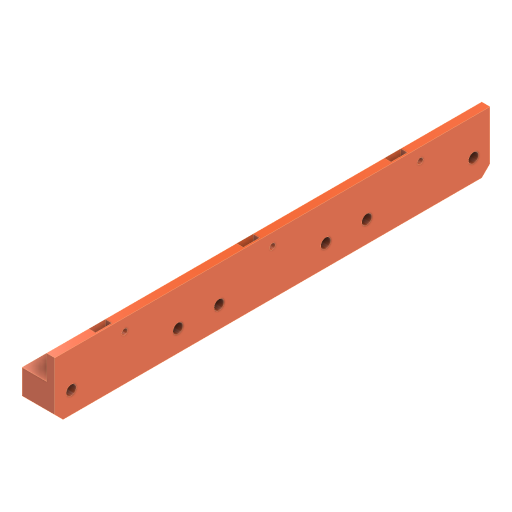
# Autodesk Inventor part: Toolhead Dock Assembly
Saved by Autodesk Inventor 2023.2 (Build 272271000, 271)
## iProperties
Created: 2023-02-06
Part Number: Toolhead Dock Assembly
Material: ABS Plastic
Document SubType Name: Modeling
Designer: remop
Density: 1.06 g/cm^3
Appearance: Smooth - Light Orange
Author: remop
Autodesk Inventor part; units mm, degrees
ref_plane "YZ Plane" through (0, 0, 0) normal (1, 0, 0) x (0, 1, 0)
ref_plane "XZ Plane" through (0, 0, 0) normal (0, 1, 0) x (-1, 0, 0)
ref_plane "XY Plane" through (0, 0, 0) normal (0, 0, 1) x (1, 0, 0)
sketch "Sketch1" plane through (0, 0, 0) normal (0, 0, 1) x (1, 0, 0)
  line L0 (0, 0) -> (0, 15)
  line L1 (0, 15) -> (5, 15)
  line L2 (5, 15) -> (5, -20)
  line L3 (5, -20) -> (-15, -20)
  line L4 (-15, -20) -> (-15, 0)
  line L5 (-15, 0) -> (0, 0)
  dimension "d0" = 15
  dimension "d1" = 5
  dimension "d2" = 35
  constraints: 12 end point, 6 perpendicular, 1 vertical
  measures "d0" distance of L0.start L0.end
  measures "d1" distance of L0.end L1.end
  measures "d2" distance of L1.end L2.end
extrude "Extrusion1" add sketch "Sketch1" along normal blind 265
sketch "Sketch2" plane through (5, -20, 0) normal (1, 0, 0) x (0, 0, -1)
  line L0 (0, 0) -> (0, 35) projected
  line L1 (0, 35) -> (-265, 35) projected
  line L2 (-265, 0) -> (-265, 35) projected
  line L3 (0, 0) -> (-265, 0) projected
  point P0 (0, 20)
  point P1 (-222.5, 27.5)
  point P2 (-132.5, 27.5)
  point P3 (-42.5, 27.5)
  point P4 (-132.5, 35)
  dimension "d5" = 90
  dimension "d6" = 90
  dimension "d7" = 7.5
  constraints: 2 horizontal alignment, 1 midpoint, 1 vertical alignment
  measures "d5" distance of point (-132.5, 27.5) point (-222.5, 27.5)
  measures "d6" distance of point (-42.5, 27.5) point (-132.5, 27.5)
  measures "d7" distance from line of L1 point (-132.5, 27.5)
hole "Hole1" at (5, 7.5, 222.5) at (5, 7.5, 132.5) at (5, 7.5, 42.5) direction (-1, 0, 0) diameter 3.5 end through all
chamfer "Chamfer1" distance 5 angle 45 2 edges at (-5, -20, 265) (-5, -20, 0)
sketch "Sketch3" plane through (-15, 0, 0) normal (-1, 0, 0) x (0, 0, 1)
  line L0 (5, -20) -> (260, -20) projected
  line L1 (265, -15) -> (260, -20) projected
  line L2 (265, 0) -> (265, -15) projected
  line L3 (5, -20) -> (0, -15) projected
  line L4 (0, 0) -> (0, -15) projected
  line L5 (0, 0) -> (265, 0) projected
  point P0 (52.5, -10)
  point P1 (132.5, -10)
  point P2 (212.5, -10)
  point P3 (132.5, -20)
  dimension "d18" = 80
  dimension "d19" = 80
  dimension "d20" = 10
  constraints: 2 horizontal alignment, 1 midpoint, 1 vertical alignment
  measures "d18" distance of point (212.5, -10) point (132.5, -10)
  measures "d19" distance of point (52.5, -10) point (132.5, -10)
  measures "d20" distance from line of L5 point (132.5, -10)
hole "Hole2" at (-15, -10, 52.5) at (-15, -10, 132.5) at (-15, -10, 212.5) direction (1, 0, 0) diameter 2.8 depth 15
sketch "Sketch4" plane through (5, 15, 265) normal (1, 0, 0) x (0, 0, -1)
  circle A0 centre (132.5, -7.5) radius 1.75 projected
  circle A1 centre (42.5, -7.5) radius 1.75 projected
  circle A2 centre (222.5, -7.5) radius 1.75 projected
  line L0 (265, -30) -> (260, -35) projected
  line L1 (265, -30) -> (265, 0) projected
  line L2 (265, 0) -> (0, 0) projected
  line L3 (0, -30) -> (0, 0) projected
  line L4 (5, -35) -> (0, -30) projected
  line L5 (260, -35) -> (5, -35) projected
  point P0 (265, -15)
  point P1 (10, -22)
  point P2 (75, -22)
  point P3 (100, -22)
  point P4 (165, -22)
  point P5 (255, -22)
  point P6 (190, -22)
  dimension "d28" = 10
  dimension "d29" = 22
  dimension "d30" = 65
  dimension "d31" = 25
  dimension "d32" = 65
  dimension "d33" = 65
  dimension "d34" = 25
  dimension "d43" = 10
  constraints: 5 horizontal alignment
  measures "d28" distance from line of L3 point (10, -22)
  measures "d29" distance from line of L2 point (10, -22)
  measures "d30" distance of point (75, -22) point (10, -22)
  measures "d31" distance of point (100, -22) point (75, -22)
  measures "d32" distance of point (165, -22) point (100, -22)
  measures "d33" distance of point (255, -22) point (190, -22)
  measures "d34" distance of point (165, -22) point (190, -22)
  measures "d43" distance from line of L1 point (255, -22)
hole "Hole3" at (5, -7, 255) at (5, -7, 190) at (5, -7, 165) at (5, -7, 100) at (5, -7, 10) at (5, -7, 75) direction (-1, 0, 0) diameter 6 end through all
sketch "Sketch5" plane through (-15, -20, 5) normal (0, -1, 0) x (1, 0, 0)
  line L0 (20, 0) -> (0, 0) projected
  line L1 (20, 0) -> (20, 255) projected
  line L2 (0, 255) -> (20, 255) projected
  line L3 (0, 0) -> (0, 255) projected
  line L4 (15, 35.75) -> (15, 39.25) projected
  line L5 (20, 39.25) -> (20, 35.75) projected
  line L6 (15, 125.75) -> (15, 129.25) projected
  line L7 (20, 129.25) -> (20, 125.75) projected
  line L8 (15, 215.75) -> (15, 219.25) projected
  line L9 (20, 219.25) -> (20, 215.75) projected
  line L10 (19, 224.25) -> (13, 224.25)
  line L11 (13, 224.25) -> (13, 234.25)
  line L12 (13, 234.25) -> (19, 234.25)
  line L13 (19, 234.25) -> (19, 224.25)
  line L14 (19, 134.25) -> (13, 134.25)
  line L15 (13, 134.25) -> (13, 144.25)
  line L16 (13, 144.25) -> (19, 144.25)
  line L17 (19, 144.25) -> (19, 134.25)
  line L18 (19, 44.25) -> (13, 44.25)
  line L19 (13, 44.25) -> (13, 54.25)
  line L20 (13, 54.25) -> (19, 54.25)
  line L21 (19, 54.25) -> (19, 44.25)
  point P0 (15, -5)
  dimension "d44" = 1
  dimension "d45" = 5
  dimension "d46" = 5
  dimension "d47" = 5
  dimension "d48" = 10
  dimension "d49" = 6
  constraints: 24 end point, 6 parallel, 4 equal length, 3 horizontal, 3 perpendicular, 2 vertical alignment
  measures "d44" distance between parallel lines of L1 L13
  measures "d45" distance from line of L6.end L14
  measures "d46" distance from line of L8.end L10
  measures "d47" distance from line of L4.end L18
  measures "d48" distance of L16.end L14.start
  measures "d49" distance of L14.start L14.end
extrude "Extrusion2" cut sketch "Sketch5" against normal through all contours L10 L11 L12 L13 | L14 L15 L16 L17 | L18 L19 L20 L21
equation "\"d6\" = d5"
equation "\"d19\" = d18"
equation "\"d32\" = d30"
equation "\"d33\" = d32"
equation "\"d34\" = d31"
equation "\"d46\" = d45"
equation "\"d47\" = d45"
body "Solid1"
